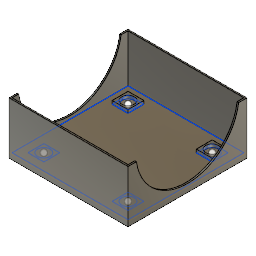
Camisa v0 (Autodesk Fusion 360 design; units mm, degrees)
Autodesk Fusion 360 part; units mm, degrees
note: some values were not read from the file. Set by a fixed rule: which sketch regions a step uses.
sketch "Sketch1" plane through (0, 0, 0) normal (0, 0, 1) x (1, 0, 0)
  line L0 (17.4335, 12.3824) -> (92.4335, 12.3824)
  line L1 (92.4335, 12.3824) -> (92.4335, 87.3824)
  line L2 (92.4335, 87.3824) -> (17.4335, 87.3824)
  line L3 (17.4335, 87.3824) -> (17.4335, 12.3824)
  dimension "d1" = 75
  dimension "d2" = 75
  constraint horizontal L0
  constraint vertical L1
  constraint horizontal L2
  constraint vertical L3
  measures "d1" distance of L0.start L0.end
  measures "d2" distance of L0.start L2.end
extrude "Extrude1" add sketch "Sketch1" along normal blind 3
sketch "Sketch2" plane through (0, 0, 0) normal (0, 0, -1) x (1, 0, 0)
  line L0 (17.4335, -12.3824) -> (17.4335, -87.3824)
  line L1 (17.4335, -87.3824) -> (92.4335, -87.3824)
  line L2 (92.4335, -87.3824) -> (92.4335, -12.3824)
  line L3 (92.4335, -12.3824) -> (17.4335, -12.3824)
  line L4 (54.6048, -60.3835) -> (54.3, -59.8366)
  spline S0 degree 3 poles (54.2649, -61.2659) (54.2437, -62.1347) (54.2025, -62.7006) (54.1599, -62.7089) knots 0 0 0 0 1 1 1 1
  line L5 (52.4329, -52.2867) -> (53.6731, -54.4165)
  line L6 (48.7322, -50.1134) -> (48.5846, -49.8647)
  line L7 (51.2198, -54.4134) -> (49.9808, -54.4123)
  line L8 (54.3, -59.8366) -> (54.2649, -61.2659)
  spline S1 degree 3 poles (49.9247, -52.3071) (49.9247, -52.2684) (49.43, -52.2411) (48.7272, -52.2411) knots 0 0 0 0 1 1 1 1
  spline S2 degree 3 poles (48.7272, -52.2411) (47.7971, -52.2411) (47.5374, -52.2216) (47.5645, -52.1536) knots 0 0 0 0 1 1 1 1
  line L9 (51.8323, -55.4838) -> (51.2198, -54.4134)
  spline S3 degree 3 poles (46.2145, -54.4103) (46.2145, -54.4557) (46.6636, -54.4824) (47.4571, -54.484) knots 0 0 0 0 1 1 1 1
  spline S4 degree 3 poles (47.5645, -52.1536) (47.5838, -52.1055) (47.8544, -51.6268) (48.1659, -51.0898) knots 0 0 0 0 1 1 1 1
  spline S5 degree 3 poles (44.9544, -52.2578) (44.9544, -52.2872) (45.4933, -52.3113) (46.152, -52.3113) knots 0 0 0 0 1 1 1 1
  spline S6 degree 3 poles (48.5846, -49.8647) (48.5033, -49.7279) (48.2192, -49.2347) (47.9532, -48.7688) knots 0 0 0 0 1 1 1 1
  line L10 (49.9808, -54.4123) -> (48.7417, -54.4113)
  line L11 (47.4571, -54.484) -> (48.6997, -54.4867)
  spline S7 degree 3 poles (53.1996, -50.952) (52.9329, -51.4108) (52.6512, -51.8987) (52.5738, -52.0364) knots 0 0 0 0 1 1 1 1
  line L12 (53.0931, -49.0969) -> (53.6845, -50.1179)
  line L13 (49.3059, -55.5517) -> (49.9121, -56.6166)
  line L14 (49.9121, -56.6166) -> (51.1785, -56.6357)
  spline S8 degree 3 poles (46.7396, -53.4358) (46.4508, -53.9326) (46.2145, -54.3711) (46.2145, -54.4103) knots 0 0 0 0 1 1 1 1
  spline S9 degree 3 poles (42.312, -52.3854) (42.1407, -51.5831) (42.1241, -51.3687) (42.1218, -49.9312) knots 0 0 0 0 1 1 1 1
  line L15 (53.6845, -50.1179) -> (53.1996, -50.952)
  line L16 (48.7417, -54.4113) -> (49.3332, -53.3922)
  spline S10 degree 3 poles (45.9005, -50.5646) (45.3801, -51.4664) (44.9544, -52.2283) (44.9544, -52.2578) knots 0 0 0 0 1 1 1 1
  line L17 (53.5649, -62.6639) -> (53.565, -62.6641)
  spline S11 degree 3 poles (47.3071, -52.4219) (47.2837, -52.4828) (47.0284, -52.939) (46.7396, -53.4358) knots 0 0 0 0 1 1 1 1
  spline S12 degree 3 poles (52.4449, -56.6045) (52.4449, -56.5768) (52.1692, -56.0725) (51.8323, -55.4838) knots 0 0 0 0 1 1 1 1
  line L18 (48.6997, -54.4867) -> (49.3059, -55.5517)
  spline S13 degree 3 poles (62.403, -54.4831) (63.1327, -54.482) (63.6456, -54.454) (63.6456, -54.4153) knots 0 0 0 0 1 1 1 1
  spline S14 degree 3 poles (62.3155, -52.2146) (62.3155, -52.2292) (61.78, -52.2411) (61.1254, -52.2411) knots 0 0 0 0 1 1 1 1
  line L19 (59.9236, -56.6514) -> (60.542, -55.5682)
  spline S15 degree 3 poles (67.7562, -49.4517) (67.8288, -51.6464) (67.4266, -53.5568) (66.4837, -55.4963) knots 0 0 0 0 1 1 1 1
  spline S16 degree 3 poles (61.9767, -48.6416) (61.7552, -49.0235) (61.4743, -49.5109) (61.3525, -49.7246) knots 0 0 0 0 1 1 1 1
  line L20 (61.1604, -54.4849) -> (62.403, -54.4831)
  line L21 (63.0541, -53.3302) -> (62.4625, -52.3111)
  line L22 (61.3525, -49.7246) -> (61.131, -50.1133)
  spline S17 degree 3 poles (64.8797, -52.2045) (64.8572, -52.1459) (64.4273, -51.3848) (63.9244, -50.5132) knots 0 0 0 0 1 1 1 1
  spline S18 degree 3 poles (58.0275, -55.4799) (57.6907, -56.0676) (57.4152, -56.5716) (57.4152, -56.5999) knots 0 0 0 0 1 1 1 1
  spline S19 degree 3 poles (61.1254, -52.2411) (60.3243, -52.2411) (59.9353, -52.2657) (59.9353, -52.3163) knots 0 0 0 0 1 1 1 1
  spline S20 degree 3 poles (63.6456, -54.4153) (63.6456, -54.379) (63.3794, -53.8907) (63.0541, -53.3302) knots 0 0 0 0 1 1 1 1
  spline S21 degree 3 poles (61.0285, -54.3022) (61.0654, -54.3984) (60.9268, -54.4113) (59.8551, -54.4113) knots 0 0 0 0 1 1 1 1
  spline S22 degree 3 poles (57.4152, -56.5999) (57.4152, -56.6282) (57.9796, -56.6514) (58.6694, -56.6514) knots 0 0 0 0 1 1 1 1
  spline S23 degree 3 poles (60.461, -53.2923) (60.7501, -53.7877) (61.0055, -54.2422) (61.0285, -54.3022) knots 0 0 0 0 1 1 1 1
  spline S24 degree 3 poles (54.9221, -56.5584) (54.9269, -56.5651) (55.2075, -56.0925) (55.5456, -55.5084) knots 0 0 0 0 1 1 1 1
  line L23 (46.1558, -45.786) -> (46.6109, -46.5694)
  line L24 (65.2684, -47.8088) -> (67.4162, -46.7988)
  spline S25 degree 3 poles (54.4007, -47.0795) (54.1176, -46.588) (53.8152, -46.0532) (53.7288, -45.891) knots 0 0 0 0 1 1 1 1
  spline S26 degree 3 poles (58.8481, -45.5732) (59.4175, -44.5818) (59.9029, -43.7711) (59.9268, -43.7717) knots 0 0 0 0 1 1 1 1
  spline S27 degree 3 poles (66.016, -43.3854) (66.4025, -44.039) (66.8976, -45.0776) (66.9485, -45.3415) knots 0 0 0 0 1 1 1 1
  line L25 (47.4695, -47.9217) -> (48.1006, -46.8437)
  spline S28 degree 3 poles (61.0036, -45.5743) (61.5718, -46.5651) (62.1138, -47.5044) (62.208, -47.6615) knots 0 0 0 0 1 1 1 1
  spline S29 degree 3 poles (64.9067, -46.4293) (63.7715, -46.964) (62.8317, -47.3906) (62.8185, -47.3773) knots 0 0 0 0 1 1 1 1
  spline S30 degree 3 poles (53.7288, -45.891) (53.5723, -45.5973) (50.7538, -40.6654) (50.225, -39.7599) knots 0 0 0 0 1 1 1 1
  spline S31 degree 3 poles (48.3147, -42.0557) (47.4954, -43.4803) (46.6746, -44.9024) (46.4905, -45.2159) knots 0 0 0 0 1 1 1 1
  line L26 (55.5951, -43.6308) -> (55.5951, -40.3302)
  spline S32 degree 3 poles (64.1373, -40.9447) (64.9892, -41.8247) (65.4368, -42.4062) (66.016, -43.3854) knots 0 0 0 0 1 1 1 1
  line L27 (54.265, -40.3302) -> (54.265, -43.6308)
  spline S33 degree 3 poles (59.976, -39.3791) (59.8988, -39.2941) (59.7686, -39.5116) (56.9265, -44.4708) knots 0 0 0 0 1 1 1 1
  line L28 (42.8668, -45.4329) -> (42.9578, -45.1794)
  spline S34 degree 3 poles (42.9578, -45.1794) (43.801, -42.8284) (45.8434, -40.3845) (48.1774, -38.9338) knots 0 0 0 0 1 1 1 1
  spline S35 degree 3 poles (63.6456, -45.7928) (63.6456, -45.7037) (60.1137, -39.5308) (59.976, -39.3791) knots 0 0 0 0 1 1 1 1
  spline S36 degree 3 poles (49.3107, -44.7692) (49.6292, -44.2212) (49.9084, -43.7723) (49.9313, -43.7717) knots 0 0 0 0 1 1 1 1
  spline S37 degree 3 poles (56.1551, -45.8359) (55.8252, -46.4388) (55.0992, -47.7043) (54.9999, -47.8495) knots 0 0 0 0 1 1 1 1
  spline S38 degree 3 poles (42.4325, -46.9238) (42.4814, -46.8448) (42.9158, -47.0237) (44.6165, -47.8231) knots 0 0 0 0 1 1 1 1
  line L29 (46.4905, -45.2159) -> (46.1558, -45.786)
  spline S39 degree 3 poles (59.9268, -43.7717) (59.9508, -43.7722) (60.4353, -44.5834) (61.0036, -45.5743) knots 0 0 0 0 1 1 1 1
  spline S40 degree 3 poles (63.2199, -46.6157) (63.454, -46.2101) (63.6456, -45.8398) (63.6456, -45.7928) knots 0 0 0 0 1 1 1 1
  spline S41 degree 3 poles (55.5456, -55.5084) (55.8837, -54.9242) (56.4436, -53.9594) (56.7897, -53.3644) knots 0 0 0 0 1 1 1 1
  spline S42 degree 3 poles (56.8117, -51.2293) (56.4776, -50.65) (56.2051, -50.1445) (56.206, -50.106) knots 0 0 0 0 1 1 1 1
  spline S43 degree 3 poles (61.7232, -51.1507) (62.049, -51.7212) (62.3155, -52.2) (62.3155, -52.2146) knots 0 0 0 0 1 1 1 1
  line L30 (57.4191, -52.2826) -> (56.8117, -51.2293)
  spline S44 degree 3 poles (59.9353, -52.3163) (59.9353, -52.3576) (60.1719, -52.7968) (60.461, -53.2923) knots 0 0 0 0 1 1 1 1
  spline S45 degree 3 poles (47.041, -47.3779) (47.0272, -47.3917) (46.0824, -46.9597) (44.9414, -46.4179) knots 0 0 0 0 1 1 1 1
  spline S46 degree 3 poles (57.5189, -47.8309) (57.6806, -47.5806) (58.2788, -46.5647) (58.8481, -45.5732) knots 0 0 0 0 1 1 1 1
  spline S47 degree 3 poles (66.9485, -45.3415) (66.9657, -45.4309) (66.5013, -45.6783) (64.9067, -46.4293) knots 0 0 0 0 1 1 1 1
  spline S48 degree 3 poles (51.149, -45.8182) (51.7958, -46.9444) (52.3648, -47.9131) (52.4133, -47.9709) knots 0 0 0 0 1 1 1 1
  spline S49 degree 3 poles (49.9313, -43.7717) (49.9542, -43.7711) (50.5021, -44.692) (51.149, -45.8182) knots 0 0 0 0 1 1 1 1
  spline S50 degree 3 poles (54.9999, -47.8495) (54.9261, -47.9575) (54.8504, -47.8602) (54.4007, -47.0795) knots 0 0 0 0 1 1 1 1
  line L31 (54.93, -43.6308) -> (55.5951, -43.6308)
  line L32 (44.9414, -46.4179) -> (42.8668, -45.4329)
  line L33 (67.4162, -46.7988) -> (67.4889, -47.1223)
  line L34 (62.208, -47.6615) -> (62.3793, -47.9472)
  line L35 (58.6694, -56.6514) -> (59.9236, -56.6514)
  line L36 (59.8551, -54.4113) -> (58.6399, -54.4113)
  line L37 (55.5946, -61.215) -> (55.594, -59.7666)
  spline S51 degree 3 poles (49.3332, -53.3922) (49.6585, -52.8317) (49.9247, -52.3434) (49.9247, -52.3071) knots 0 0 0 0 1 1 1 1
  spline S52 degree 3 poles (51.1785, -56.6357) (51.875, -56.6462) (52.4449, -56.6321) (52.4449, -56.6045) knots 0 0 0 0 1 1 1 1
  spline S53 degree 3 poles (46.152, -52.3113) (47.2148, -52.3113) (47.3448, -52.3238) (47.3071, -52.4219) knots 0 0 0 0 1 1 1 1
  line L38 (60.542, -55.5682) -> (61.1604, -54.4849)
  line L39 (56.7897, -53.3644) -> (57.4191, -52.2826)
  spline S54 degree 3 poles (56.2601, -62.6626) (55.9521, -62.6957) (55.6764, -62.7095) (55.6476, -62.6932) knots 0 0 0 0 1 1 1 1
  line L40 (52.5738, -52.0364) -> (52.4329, -52.2867)
  line L41 (48.1659, -51.0898) -> (48.7322, -50.1134)
  line L42 (55.594, -59.7666) -> (55.2747, -60.3256)
  spline S55 degree 3 poles (55.6476, -62.6932) (55.6187, -62.6768) (55.5948, -62.0117) (55.5946, -61.215) knots 0 0 0 0 1 1 1 1
  spline S56 degree 3 poles (66.4837, -55.4963) (64.5596, -59.4539) (60.6573, -62.1892) (56.2601, -62.6626) knots 0 0 0 0 1 1 1 1
  spline S57 degree 3 poles (46.793, -48.8731) (46.8225, -48.9017) (46.4208, -49.6629) (45.9005, -50.5646) knots 0 0 0 0 1 1 1 1
  spline S58 degree 3 poles (55.2747, -60.3256) (55.0991, -60.633) (54.9451, -60.8948) (54.9325, -60.9074) knots 0 0 0 0 1 1 1 1
  line L43 (58.6399, -54.4113) -> (58.0275, -55.4799)
  line L44 (62.4625, -52.3111) -> (63.6916, -52.3111)
  line L45 (61.131, -50.1133) -> (61.7232, -51.1507)
  spline S59 degree 3 poles (48.1006, -46.8437) (48.4477, -46.2508) (48.9922, -45.3173) (49.3107, -44.7692) knots 0 0 0 0 1 1 1 1
  spline S60 degree 3 poles (56.9265, -44.4708) (56.6287, -44.9906) (56.2815, -45.6049) (56.1551, -45.8359) knots 0 0 0 0 1 1 1 1
  spline S61 degree 3 poles (62.8185, -47.3773) (62.8052, -47.364) (62.9858, -47.0213) (63.2199, -46.6157) knots 0 0 0 0 1 1 1 1
  spline S62 degree 3 poles (42.2454, -47.6893) (42.3148, -47.3225) (42.399, -46.9781) (42.4325, -46.9238) knots 0 0 0 0 1 1 1 1
  line L46 (54.265, -43.6308) -> (54.93, -43.6308)
  spline S63 degree 3 poles (46.6109, -46.5694) (46.8612, -47.0003) (47.0548, -47.3641) (47.041, -47.3779) knots 0 0 0 0 1 1 1 1
  line L47 (55.5951, -40.3302) -> (55.5951, -37.0296)
  spline S64 degree 3 poles (58.9875, -37.6867) (61.0337, -38.3679) (62.6051, -39.3621) (64.1373, -40.9447) knots 0 0 0 0 1 1 1 1
  spline S65 degree 3 poles (48.1774, -38.9338) (49.7721, -37.9425) (51.9571, -37.2076) (53.7118, -37.0723) knots 0 0 0 0 1 1 1 1
  line L48 (53.7118, -37.0723) -> (54.265, -37.0296)
  line L49 (54.265, -37.0296) -> (54.265, -40.3302)
  spline S66 degree 3 poles (56.1483, -37.0723) (56.9501, -37.1341) (58.029, -37.3676) (58.9875, -37.6867) knots 0 0 0 0 1 1 1 1
  line L50 (55.5951, -37.0296) -> (56.1483, -37.0723)
  spline S67 degree 3 poles (50.225, -39.7599) (50.0154, -39.401) (49.9296, -39.3064) (49.8757, -39.3748) knots 0 0 0 0 1 1 1 1
  spline S68 degree 3 poles (49.8757, -39.3748) (49.8363, -39.4247) (49.1339, -40.6311) (48.3147, -42.0557) knots 0 0 0 0 1 1 1 1
  spline S69 degree 3 poles (63.6916, -52.3111) (64.7634, -52.3111) (64.9154, -52.2975) (64.8797, -52.2045) knots 0 0 0 0 1 1 1 1
  spline S70 degree 3 poles (63.9244, -50.5132) (63.4214, -49.6416) (63.0348, -48.9039) (63.0652, -48.8737) knots 0 0 0 0 1 1 1 1
  line L51 (62.3793, -47.9472) -> (61.9767, -48.6416)
  spline S71 degree 3 poles (53.565, -62.6641) (51.8513, -62.4724) (50.0296, -61.883) (48.5711, -61.0484) knots 0 0 0 0 1 1 1 1
  spline S72 degree 3 poles (56.206, -50.106) (56.2081, -50.0238) (57.0941, -48.4884) (57.5189, -47.8309) knots 0 0 0 0 1 1 1 1
  spline S73 degree 3 poles (53.6731, -54.4165) (54.3553, -55.588) (54.9173, -56.5518) (54.9221, -56.5584) knots 0 0 0 0 1 1 1 1
  spline S74 degree 3 poles (63.0652, -48.8737) (63.0956, -48.8435) (64.0871, -48.3644) (65.2684, -47.8088) knots 0 0 0 0 1 1 1 1
  spline S75 degree 3 poles (42.1218, -49.9312) (42.1199, -48.6988) (42.1467, -48.211) (42.2454, -47.6893) knots 0 0 0 0 1 1 1 1
  spline S76 degree 3 poles (54.1599, -62.7089) (54.1214, -62.7165) (53.8537, -62.6962) (53.5649, -62.6639) knots 0 0 0 0 1 1 1 1
  spline S77 degree 3 poles (52.4133, -47.9709) (52.4619, -48.0286) (52.7678, -48.5353) (53.0931, -49.0969) knots 0 0 0 0 1 1 1 1
  spline S78 degree 3 poles (48.5711, -61.0484) (45.3506, -59.2055) (43.1041, -56.0961) (42.312, -52.3854) knots 0 0 0 0 1 1 1 1
  spline S79 degree 3 poles (67.4889, -47.1223) (67.6705, -47.9293) (67.7202, -48.3629) (67.7562, -49.4517) knots 0 0 0 0 1 1 1 1
  line L52 (47.9532, -48.7688) -> (47.4695, -47.9217)
  spline S80 degree 3 poles (44.6165, -47.8231) (45.7842, -48.372) (46.7636, -48.8445) (46.793, -48.8731) knots 0 0 0 0 1 1 1 1
  spline S81 degree 3 poles (54.9325, -60.9074) (54.9199, -60.92) (54.7725, -60.6843) (54.6048, -60.3835) knots 0 0 0 0 1 1 1 1
  point P0 (-15.495, 55.0698)
extrude "Extrude2" cut sketch "Sketch2" against normal blind 1.5 contours L4 S0 L5 L6 L7 L8 S1 S2 L9 S3 S4 S5 S6 L10 L11 S7 L12 L13 L14 S8 S9 L15 L16 S10 S11 S12 L18 S13 S14 L19 S15 S16 L20 L21 L22 S17 S18 S19 S20 S21 S22 S23 S24 L24 S26 L25 S28 S36 S38 S39 S41 S42 S43 L30 S44 S46 S48 S49 L33 L34 L35 L36 L37 S51 S52 S53 L38 L39 S54 L40 L41 L42 S55 S56 S57 S58 L43 L44 L45 S59 S62 S69 S70 L51 S71 S72 S73 S74 S75 S76 S77 S78 S79 L52 S80 S81 | L23 S25 S27 S29 S30 S31 L26 S32 L27 S33 L28 S34 S35 S37 L29 S40 S45 S47 S50 L31 L32 S60 S61 L46 S63 L47 S64 S65 L48 L49 S66 L50 S67 S68
sketch "Sketch4" plane through (0, 0, 3) normal (0, 0, 1) x (-1, 0, 0)
  line L0 (-17.4335, -87.3824) -> (-17.4335, -12.3824)
  line L1 (-17.4335, -12.3824) -> (-92.4335, -12.3824)
  line L2 (-92.4335, -12.3824) -> (-92.4335, -87.3824)
  line L3 (-92.4335, -87.3824) -> (-17.4335, -87.3824)
  line L4 (-18.4335, -13.3824) -> (-91.4335, -13.3824)
  line L5 (-91.4335, -13.3824) -> (-91.4335, -86.3824)
  line L6 (-91.4335, -86.3824) -> (-18.4335, -86.3824)
  line L7 (-18.4335, -86.3824) -> (-18.4335, -13.3824)
  line L8 (-23.4335, -71.3824) -> (-33.4335, -71.3824)
  line L9 (-33.4335, -71.3824) -> (-33.4335, -81.3824)
  line L10 (-33.4335, -81.3824) -> (-23.4335, -81.3824)
  line L11 (-23.4335, -81.3824) -> (-23.4335, -71.3824)
  circle A0 centre (-28.4335, -76.3824) radius 4
  line L12 (-23.4335, -71.3824) -> (-33.4335, -71.3824)
  line L13 (-33.4335, -71.3824) -> (-33.4335, -81.3824)
  line L14 (-23.4335, -81.3824) -> (-23.4335, -71.3824)
  line L15 (-33.4335, -81.3824) -> (-23.4335, -81.3824)
  circle A1 centre (-28.4335, -76.3824) radius 4
  line L16 (-76.4335, -18.3824) -> (-86.4335, -18.3824)
  line L17 (-86.4335, -18.3824) -> (-86.4335, -28.3824)
  line L18 (-76.4335, -28.3824) -> (-76.4335, -18.3824)
  line L19 (-86.4335, -28.3824) -> (-76.4335, -28.3824)
  circle A2 centre (-81.4335, -23.3824) radius 4
  line L20 (-86.4335, -71.3824) -> (-86.4335, -81.3824)
  line L21 (-86.4335, -81.3824) -> (-76.4335, -81.3824)
  circle A3 centre (-81.4335, -76.3824) radius 4
  line L22 (-76.4335, -81.3824) -> (-76.4335, -71.3824)
  line L23 (-76.4335, -71.3824) -> (-86.4335, -71.3824)
  line L24 (-23.4335, -18.3824) -> (-33.4335, -18.3824)
  line L25 (-23.4335, -28.3824) -> (-23.4335, -18.3824)
  line L26 (-33.4335, -28.3824) -> (-23.4335, -28.3824)
  line L27 (-33.4335, -18.3824) -> (-33.4335, -28.3824)
  circle A4 centre (-28.4335, -23.3824) radius 4
  dimension "d11" = 8
  dimension "d16" = 8
  dimension "d17" = 8
  dimension "d18" = 8
  dimension "d19" = 8
  constraint horizontal L4
  constraint vertical L5
  constraint horizontal L6
  constraint vertical L7
  constraint horizontal L8
  constraint vertical L9
  constraint horizontal L10
  constraint vertical L11
  constraint horizontal L12
  constraint vertical L13
  constraint horizontal L15
  constraint vertical L14
  constraint horizontal L16
  constraint vertical L17
  constraint horizontal L19
  constraint vertical L18
  constraint horizontal L23
  constraint vertical L20
  constraint horizontal L21
  constraint vertical L22
  constraint horizontal L24
  constraint vertical L27
  constraint horizontal L26
  constraint vertical L25
  measures "d11" diameter of A0
  measures "d16" diameter of A1
  measures "d17" diameter of A2
  measures "d18" diameter of A3
  measures "d19" diameter of A4
extrude "Extrude4" add sketch "Sketch4" along normal blind 30 contours L0 L1 L2 L3
extrude "Extrude3" add sketch "Sketch4" along normal blind 2 contours L8 L9 L10 L11 L12 L13 L14 L15 | L16 L17 L18 L19 | L20 L21 L22 L23 | L24 L25 L26 L27
sketch "Sketch5" plane through (17.4335, 0, 0) normal (-1, 0, 0) x (0, -1, 0)
  line L0 (-87.3824, 0) -> (-12.3824, 0)
  line L1 (-12.3824, 0) -> (-12.3824, 33)
  line L2 (-12.3824, 33) -> (-87.3824, 33)
  line L3 (-87.3824, 33) -> (-87.3824, 0)
  line L4 (-12.3824, 0) -> (-12.3824, 75)
  line L5 (-87.3824, 0) -> (-87.3824, 75)
  line L6 (-87.3824, 75) -> (-12.3824, 75)
  circle A0 centre (-49.8824, 37.5) radius 32.5
  dimension "d24" = 75
  dimension "d25" = 75
  dimension "d26" = 65
  constraint coincident L0.end L1.start
  constraint perpendicular L0 L4
  constraint coincident L0.start L3.end
  constraint perpendicular L2 L5
  measures "d24" distance of L0.end L4.end
  measures "d25" distance of L0.start L5.end
  measures "d26" diameter of A0
extrude "Extrude5" cut sketch "Sketch5" against normal blind 1 contours L2 A0 picked at (-51.4283, 23.7775)
sketch "Sketch6" plane through (92.4335, 0, 0) normal (1, 0, 0) x (0, 1, 0)
  line L0 (12.3824, 0) -> (87.3824, 0)
  line L1 (87.3824, 0) -> (87.3824, 33)
  line L2 (87.3824, 33) -> (12.3824, 33)
  line L3 (12.3824, 33) -> (12.3824, 0)
  line L4 (12.3824, 0) -> (12.3824, 75)
  line L5 (12.3824, 75) -> (87.3824, 75)
  line L6 (87.3824, 75) -> (87.3824, 0)
  circle A0 centre (49.8824, 37.5) radius 32.5
  dimension "d29" = 75
  dimension "d30" = 75
  dimension "d31" = 65
  constraint coincident L0.start L3.end
  constraint perpendicular L0 L4
  constraint perpendicular L3 L5
  constraint coincident L0.end L1.start
  measures "d29" distance of L0.start L4.end
  measures "d30" distance of L4.end L5.end
  measures "d31" diameter of A0
extrude "Extrude6" cut sketch "Sketch6" against normal blind 1 contours L2 A0 picked at (48.3365, 23.7775)
